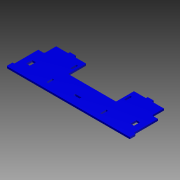
# Autodesk Inventor part: OpenROV 2_3 Dev Bulkhead
Saved by Autodesk Inventor 2012 (Build 160160000, 160)
## iProperties
Created: 2011-09-23
Part Number: OpenROV 2_3 Dev Bulkhead
Document SubType Name: Modeling
Designer: user
Density: 1 g/cm^3
Material: Default
Author: user
Autodesk Inventor part; units mm, degrees
ref_plane "YZ Plane" through (0, 0, 0) normal (1, 0, 0) x (0, 1, 0)
ref_plane "XZ Plane" through (0, 0, 0) normal (0, 1, 0) x (-1, 0, 0)
ref_plane "XY Plane" through (0, 0, 0) normal (0, 0, 1) x (1, 0, 0)
sketch "Sketch1" plane through (0, 0, 0) normal (0, 0, 1) x (1, 0, 0)
  line L0 (-40, 0) -> (-40, -29)
  line L1 (-39, -30) -> (39, -30)
  line L2 (40, -29) -> (40, 0)
  line L3 (100, -60) -> (102, -60)
  line L4 (103, -61) -> (103, -69)
  line L5 (102, -70) -> (-102, -70)
  line L6 (-103, -69) -> (-103, -61)
  line L7 (-102, -60) -> (-100, -60)
  line L8 (-60, 0) -> (-60, 3)
  line L9 (-60, 3) -> (-70, 3)
  line L10 (-70, 3) -> (-70, 0)
  line L11 (-90, 0) -> (-70, 0)
  line L12 (-60, 0) -> (-40, 0)
  line L13 (70, 0) -> (70, 3)
  line L14 (70, 3) -> (60, 3)
  line L15 (60, 3) -> (60, 0)
  line L16 (40, 0) -> (60, 0)
  line L17 (70, 0) -> (90, 0)
  arc A0 (-103, -69) -> (-102, -70) centre (-102, -69) ccw
  arc A1 (102, -70) -> (103, -69) centre (102, -69) ccw
  arc A2 (39, -30) -> (40, -29) centre (39, -29) ccw
  arc A3 (-40, -29) -> (-39, -30) centre (-39, -29) ccw
  line L18 (-90, -40) -> (-84, -40)
  line L19 (-84, -40) -> (-84, -50)
  line L20 (90, -40) -> (84, -40)
  line L21 (84, -40) -> (84, -50)
  line L22 (-43.5, -10) -> (-46.5, -10)
  line L23 (-46.5, -10) -> (-46.5, -20)
  line L24 (-46.5, -20) -> (-43.5, -20)
  line L25 (-43.5, -20) -> (-43.5, -10)
  line L26 (43.5, -10) -> (46.5, -10)
  line L27 (46.5, -10) -> (46.5, -20)
  line L28 (46.5, -20) -> (43.5, -20)
  line L29 (43.5, -20) -> (43.5, -10)
  line L30 (-46.5, -50) -> (-43.5, -50)
  line L31 (-43.5, -50) -> (-43.5, -60)
  line L32 (-43.5, -60) -> (-46.5, -60)
  line L33 (-46.5, -60) -> (-46.5, -50)
  line L34 (43.5, -50) -> (46.5, -50)
  line L35 (46.5, -50) -> (46.5, -60)
  line L36 (46.5, -60) -> (43.5, -60)
  line L37 (43.5, -60) -> (43.5, -50)
  line L38 (-5, -53) -> (5, -53)
  line L39 (5, -53) -> (5, -56)
  line L40 (5, -56) -> (-5, -56)
  line L41 (-5, -56) -> (-5, -53)
  line L42 (-100, -60) -> (-100, -20)
  line L43 (-100, -20) -> (-92, -20)
  line L44 (-90, -40) -> (-90, -50)
  line L45 (90, -40) -> (90, -50)
  line L46 (90, -50) -> (84, -50)
  line L47 (100, -60) -> (100, -20)
  line L48 (100, -20) -> (92, -20)
  line L49 (90, -18) -> (90, 0)
  line L50 (-90, 0) -> (-90, -18)
  arc A4 (-92, -20) -> (-90, -18) centre (-92, -18) ccw
  arc A5 (90, -18) -> (92, -20) centre (92, -18) ccw
  line L51 (-90, -50) -> (-84, -50)
  arc A6 (-102, -60) -> (-103, -61) centre (-102, -61) ccw
  arc A7 (103, -61) -> (102, -60) centre (102, -61) ccw
  point P0 (0, 0)
  point P1 (-40, -30)
  point P2 (40, -30)
  point P3 (103, -60)
  point P4 (103, -70)
  point P5 (-103, -70)
  point P6 (-103, -60)
  point P7 (-90, -20)
  point P8 (90, -20)
  dimension "d0" = 80
  dimension "d1" = 30
  dimension "d2" = 50
  dimension "d5" = 10
  dimension "d7" = 10
  dimension "d10" = 50
  dimension "d13" = 3
  dimension "d14" = 3
  dimension "d15" = 3
  dimension "d16" = 10
  dimension "d18" = 10
  dimension "d20" = 3
  dimension "d21" = 40
  dimension "d22" = 206
  dimension "d23" = 30
  dimension "d24" = 40
  dimension "d27" = 1
  dimension "d28" = 10
  dimension "d29" = 6
  dimension "d31" = 40
  dimension "d32" = 10
  dimension "d33" = 6
  dimension "d35" = 40
  dimension "d39" = 10
  dimension "d40" = 3
  dimension "d41" = 10
  dimension "d42" = 3
  dimension "d44" = 10
  dimension "d45" = 10
  dimension "d50" = 3
  dimension "d51" = 10
  dimension "d52" = 10
  dimension "d54" = 3
  dimension "d55" = 10
  dimension "d56" = 10
  dimension "d60" = 10
  dimension "d61" = 3
  dimension "d62" = 17
  dimension "d66" = 40
  dimension "d67" = 40
  dimension "d71" = 3.5
  dimension "d72" = 3.5
  dimension "d73" = 3.5
  dimension "d74" = 3.5
  dimension "d77" = 20
  dimension "d78" = 20
  dimension "d79" = 10
  dimension "d80" = 10
  dimension "d81" = 2
  dimension "d82" = 10
  dimension "d84" = 50
  dimension "d85" = 20
  dimension "d86" = 20
  dimension "d87" = 60
  dimension "d88" = 5
  dimension "d91" = 1
  constraints: 104 end point, 25 parallel, 16 point on circle, 16 point on line, 16 tangent, 14 perpendicular, 9 horizontal, 8 centre point, 5 equal radius, 4 collinear
  measures "d0" distance of point (-40, -30) point (40, -30)
  measures "d1" distance of point (40, -30) L2.end
  measures "d2" distance of L2.end L17.end
  measures "d5" distance of point (103, -60) point (103, -70)
  measures "d7" distance of point (-103, -70) point (-103, -60)
  measures "d10" distance of L11.start L0.start
  measures "d13" distance of L3.start point (103, -60)
  measures "d14" distance of point (-103, -60) L7.end
  measures "d15" distance between parallel lines of L9 L11
  measures "d16" distance of L8.end L9.end
  measures "d18" distance of L13.end L14.end
  measures "d20" distance between parallel lines of L17 L14
  measures "d21" distance between parallel lines of L5 L1
  measures "d22" distance of point (103, -70) point (-103, -70)
  measures "d23" distance from line of point (0, 0) L1
  measures "d24" distance from line of point (0, 0) L2
  measures "d27" radius of A0
  measures "d28" distance of L18.end L19.end
  measures "d29" distance of L18.start L18.end
  measures "d31" distance between parallel lines of L12 L18
  measures "d32" distance of L20.end L21.end
  measures "d33" distance of L20.start L20.end
  measures "d35" distance between parallel lines of L16 L20
  measures "d39" distance of L24.end L22.start
  measures "d40" distance of L23.end L24.end
  measures "d41" distance between parallel lines of L12 L22
  measures "d42" distance of L26.start L26.end
  measures "d44" distance of L26.end L27.end
  measures "d45" distance between parallel lines of L16 L26
  measures "d50" distance of L31.end L32.end
  measures "d51" distance of L32.end L30.start
  measures "d52" distance between parallel lines of L5 L32
  measures "d54" distance of L35.end L36.end
  measures "d55" distance of L34.end L35.end
  measures "d56" distance between parallel lines of L5 L36
  measures "d60" distance of L39.end L40.end
  measures "d61" distance of L38.end L39.end
  measures "d62" distance between parallel lines of L5 L38
  measures "d66" distance of L11.start L18.start
  measures "d67" distance of L20.start L17.end
  measures "d71" distance between parallel lines of L2 L29
  measures "d72" distance between parallel lines of L0 L25
  measures "d73" distance between parallel lines of L0 L31
  measures "d74" distance between parallel lines of L37 L2
  measures "d77" distance between parallel lines of L11 L43
  measures "d78" distance of point (90, -20) L17.end
  measures "d79" distance of L47.end point (90, -20)
  measures "d80" distance of L42.end point (-90, -20)
  measures "d81" radius of A4
  measures "d82" distance between parallel lines of L42 L44
  measures "d84" distance between parallel lines of L5 L43
  measures "d85" distance between parallel lines of L50 L10
  measures "d86" distance between parallel lines of L49 L13
  measures "d87" distance from line of L15 point (0, 0)
  measures "d88" distance from line of point (0, 0) L41
  measures "d91" radius of A6
extrude "Extrusion7" add sketch "Sketch1" along normal blind 3
body "Solid7"
